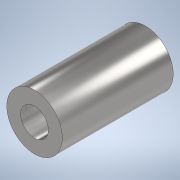
# Autodesk Inventor part: motor-tija prindere
Saved by Autodesk Inventor 2021.2 (Build 252289000, 289)
## iProperties
Created: 2024-04-21
Part Number: motor-tija prindere
Material: Stainless Steel
Document SubType Name: Modeling
Designer: cioba
Density: 8 g/cm^3
Appearance: Semi-Polished
Author: cioba
Autodesk Inventor part; units mm, degrees
ref_plane "YZ Plane" through (0, 0, 0) normal (1, 0, 0) x (0, 1, 0)
ref_plane "XZ Plane" through (0, 0, 0) normal (0, 1, 0) x (-1, 0, 0)
ref_plane "XY Plane" through (0, 0, 0) normal (0, 0, 1) x (1, 0, 0)
sketch "Sketch1" plane through (0, 0, 0) normal (0, 0, 1) x (1, 0, 0)
  circle A0 centre (-0.6511, 0.9036) radius 2.5
  circle A1 centre (-0.6511, 0.9036) radius 5
  point P0 (0, 0)
  dimension "d2" = 20
  constraints: 2 centre point, 1 coincident
extrude "Extrusion1" add sketch "Sketch1" against normal blind 20
body "Solid1"
